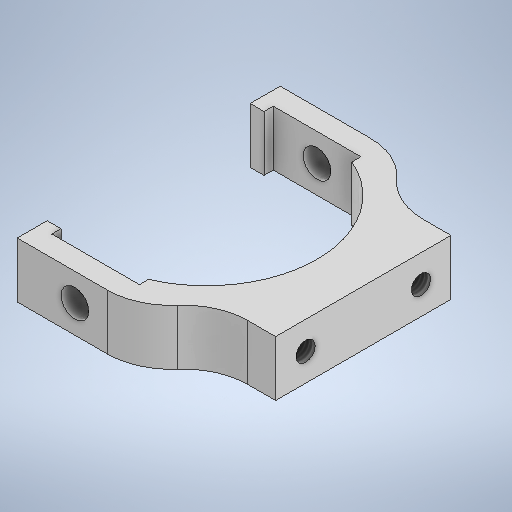
# Autodesk Inventor part: 102 new
Saved by Autodesk Inventor 2025.1 (Build 291241000, 241)
## iProperties
Created: 2024-09-04
Part Number: 102 new
Material: Generisch
Document SubType Name: Modeling
Designer: ffogue
Density: 1 g/cm^3
Appearance: Vorgabe
Author: ffogue
Autodesk Inventor part; units mm, degrees
note: some values were not read from the file. Chosen so that the rebuilt part matches the saved one: direction of "Hole2".
ref_plane "YZ Plane" through (0, 0, 0) normal (1, 0, 0) x (0, 1, 0)
ref_plane "XZ Plane" through (0, 0, 0) normal (0, 1, 0) x (-1, 0, 0)
ref_plane "XY Plane" through (0, 0, 0) normal (0, 0, 1) x (1, 0, 0)
sketch "Sketch1" plane through (0, 0, 0) normal (0, 0, 1) x (1, 0, 0)
  arc A0 (9.5, -22.0397) -> (9.5, 22.0397) centre (0, 0) ccw
  line L0 (-9.5, 22) -> (-9.5, -22) construction
  line L1 (9.5, 22.0397) -> (9.5, -22.0397) construction
  line L2 (9.5, 22.0397) -> (9.5, 24)
  line L3 (9.5, 24) -> (-9.5, 24)
  line L4 (-9.5, 24) -> (-9.5, 22)
  line L5 (-9.5, 22) -> (-12.5, 22)
  line L6 (-12.5, 22) -> (-12.5, 28.5)
  arc A1 (17.5089, 23.75) -> (28.0178, 19) centre (28.0178, 33) ccw
  line L7 (28.0178, 19) -> (34.0178, 19)
  line L8 (34.0178, 19) -> (34.0178, -19)
  line L9 (9.5, -22.0397) -> (9.5, -24)
  line L10 (9.5, -24) -> (-9.5, -24)
  line L11 (-9.5, -24) -> (-9.5, -22)
  line L12 (-12.5, -22) -> (-12.5, -28.5)
  line L13 (-9.5, -22) -> (-12.5, -22)
  arc A2 (28.0178, -19) -> (17.5089, -23.75) centre (28.0178, -33) ccw
  line L14 (28.0178, -19) -> (34.0178, -19)
  line L15 (-12.5, 28.5) -> (7, 28.5)
  arc A3 (17.5089, 23.75) -> (7, 28.5) centre (7, 14.5) ccw
  line L16 (-12.5, -28.5) -> (7, -28.5)
  arc A4 (7, -28.5) -> (17.5089, -23.75) centre (7, -14.5) ccw
  point P0 (9.5, 0)
  point P1 (0, -24)
  point P2 (0, 24)
  point P3 (-2.75, 28.5)
  point P4 (-2.75, -28.5)
  dimension "d0" = 48
  dimension "d1" = 9.5
  dimension "d2" = 9.5
  dimension "d3" = 38
  dimension "d4" = 19
  dimension "d7" = 14
  dimension "d8" = 14
  dimension "d9" = 14
  dimension "d10" = 7
  dimension "d11" = 14
  dimension "d12" = 7
  dimension "d13" = 12.5
  dimension "d14" = 12.5
  dimension "d15" = 4.5
  dimension "d16" = 4.5
  dimension "d17" = 2
  dimension "d18" = 2
  dimension "d19" = 24
  dimension "d20" = 24
  dimension "d21" = 6
  constraints: 35 end point, 10 point on circle, 6 perpendicular, 6 tangent, 5 centre point, 5 midpoint, 4 horizontal, 4 vertical, 2 parallel, 1 coincident, 1 point on line
  measures "d0" diameter of A0
  measures "d1" distance from line of point (0, 0) L0
  measures "d2" distance of point (9.5, 0) point (0, 0)
  measures "d3" distance of L7.end L8.end
  measures "d4" distance from line of point (9.5, 0) L7
  measures "d7" radius of A1
  measures "d8" radius of A2
  measures "d9" radius of A3
  measures "d10" horizontal distance of point (0, -24) A3.centre
  measures "d11" radius of A4
  measures "d12" horizontal distance of point (0, -24) A4.centre
  measures "d13" distance from line of L12 point (0, -24)
  measures "d14" distance from line of L6 point (0, 24)
  measures "d15" distance from line of L3 point (-2.75, 28.5)
  measures "d16" distance from line of point (-2.75, -28.5) L10
  measures "d17" distance between parallel lines of L10 L13
  measures "d18" distance between parallel lines of L5 L3
  measures "d19" distance from line of point (0, 0) L10
  measures "d20" distance from line of point (0, 0) L3
  measures "d21" distance of L7.start L7.end
extrude "Extrusion1" add sketch "Sketch1" along normal mid plane 12
sketch "Sketch2" plane through (34.0178, -19, 6) normal (1, 0, 0) x (0, 0, -1)
  point P0 (6, 19)
  point P1 (6, 31.5)
  point P2 (6, 6.5)
  dimension "d31" = 25
  dimension "d32" = 12.5
  constraints: 2 vertical alignment
  measures "d31" distance of point (6, 6.5) point (6, 31.5)
  measures "d32" distance of point (6, 19) point (6, 31.5)
hole "Hole1" at (34.0178, 12.5, 0) at (34.0178, -12.5, 0) direction (-1, 0, 0) diameter 4.134 end through all thread size "M5x0.8" class "6H" standard "ISO Metric profile"
sketch "Sketch3" plane through (-12.5, 28.5, 6) normal (0, 1, 0) x (1, 0, 0)
  line L0 (0, 12) -> (0, 0) projected
  point P0 (12.5, 6)
  point P1 (12.5, 6)
  point P2 (0, 6)
  point P3 (0, 6)
  dimension "d40" = 12.5
  constraints: 3 horizontal alignment, 2 midpoint
  measures "d40" distance from line of L0 point (12.5, 6)
hole "Hole2" at (0, 28.5, 0) direction (0, -1, 0) diameter 6 depth 4.5
mirror "Mirror1" about plane through (0, 0, 0) normal (0, 1, 0) of "Hole2"
equation "\"d4\" = 0.5 * d3"
equation "\"d7\" = d5"
equation "\"d8\" = d5"
equation "\"d12\" = d10"
equation "\"d14\" = d13"
equation "\"d16\" = d15"
equation "\"d20\" = d19"
equation "\"d32\" = 0.5 * d31"
equation "\"d5\" = 14"
body "Solid1"
